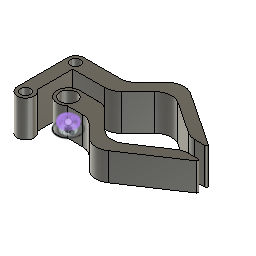
claw (Autodesk Fusion 360 design; units mm, degrees)
Autodesk Fusion 360 part; units mm, degrees
sketch "Sketch1" plane through (0, 0, 0) normal (0, 0, 1) x (1, 0, 0)
  circle A0 centre (0, 0) radius 1.75
  circle A1 centre (1.6986, -0.4211) radius 0.275
  circle A2 centre (0, 0) radius 4
  circle A3 centre (1.723, 0.3062) radius 0.275
  circle A4 centre (1.4495, 0.9805) radius 0.275
  circle A5 centre (0.9254, 1.4853) radius 0.275
  circle A6 centre (0.2412, 1.7333) radius 0.275
  circle A7 centre (-0.4846, 1.6816) radius 0.275
  circle A8 centre (-1.1267, 1.3391) radius 0.275
  circle A9 centre (-1.5739, 0.765) radius 0.275
  circle A10 centre (-1.749, 0.0587) radius 0.275
  circle A11 centre (-1.6217, -0.6577) radius 0.275
  circle A12 centre (-1.214, -1.2605) radius 0.275
  circle A13 centre (-0.5963, -1.6453) radius 0.275
  circle A14 centre (0.1244, -1.7456) radius 0.275
  circle A15 centre (0.8237, -1.5441) radius 0.275
  circle A16 centre (1.3805, -1.0756) radius 0.275
  dimension "d1" = 3.5
  dimension "d2" = 0.55
  dimension "d3" = 8
  dimension "d5" = 360
  constraint coincident A0.centre A2.centre
  constraint coincident A0 A1.centre
  measures "d1" diameter of A0
  measures "d2" diameter of A1
  measures "d3" diameter of A2
extrude "Extrude1" add sketch "Sketch1" along normal blind 2.25 makes body 1
sketch "Sketch2" plane through (0, 0, 2.25) normal (0, 0, 1) x (-1, 0, 0)
  arc A0 (-1.5319, 0.846) -> (-1.6116, 0.682) centre (0, 0) ccw
  arc A1 (-1.1949, 1.2785) -> (-1.5319, 0.846) centre (-1.3805, 1.0756) ccw
  arc A2 (-1.0554, 1.396) -> (-1.1949, 1.2785) centre (0, 0) ccw
  arc A3 (-0.5716, 1.654) -> (-1.0554, 1.396) centre (-0.8237, 1.5441) ccw
  arc A4 (-0.3963, 1.7045) -> (-0.5716, 1.654) centre (0, 0) ccw
  arc A5 (0.1506, 1.7435) -> (-0.3963, 1.7045) centre (-0.1244, 1.7456) ccw
  arc A6 (0.3312, 1.7184) -> (0.1506, 1.7435) centre (0, 0) ccw
  arc A7 (0.8467, 1.5315) -> (0.3312, 1.7184) centre (0.5963, 1.6453) ccw
  arc A8 (1.0015, 1.4351) -> (0.8467, 1.5315) centre (0, 0) ccw
  arc A9 (1.3964, 1.0547) -> (1.0015, 1.4351) centre (1.214, 1.2605) ccw
  arc A10 (1.4986, 0.9037) -> (1.3964, 1.0547) centre (0, 0) ccw
  arc A11 (1.7047, 0.3956) -> (1.4986, 0.9037) centre (1.6217, 0.6577) ccw
  arc A12 (1.7366, 0.216) -> (1.7047, 0.3956) centre (0, 0) ccw
  arc A13 (1.7182, -0.332) -> (1.7366, 0.216) centre (1.749, -0.0587) ccw
  arc A14 (1.6743, -0.509) -> (1.7182, -0.332) centre (0, 0) ccw
  arc A15 (1.4346, -1.0022) -> (1.6743, -0.509) centre (1.5739, -0.765) ccw
  arc A16 (1.3225, -1.146) -> (1.4346, -1.0022) centre (0, 0) ccw
  arc A17 (0.903, -1.499) -> (1.3225, -1.146) centre (1.1267, -1.3391) ccw
  arc A18 (0.7421, -1.5849) -> (0.903, -1.499) centre (0, 0) ccw
  arc A19 (0.2152, -1.7367) -> (0.7421, -1.5849) centre (0.4846, -1.6816) ccw
  arc A20 (0.0333, -1.7497) -> (0.2152, -1.7367) centre (0, 0) ccw
  arc A21 (-0.5098, -1.6741) -> (0.0333, -1.7497) centre (-0.2412, -1.7333) ccw
  arc A22 (-0.6812, -1.612) -> (-0.5098, -1.6741) centre (0, 0) ccw
  arc A23 (-1.1466, -1.322) -> (-0.6812, -1.612) centre (-0.9254, -1.4853) ccw
  arc A24 (-1.278, -1.1955) -> (-1.1466, -1.322) centre (0, 0) ccw
  arc A25 (-1.5852, -0.7414) -> (-1.278, -1.1955) centre (-1.4495, -0.9805) ccw
  arc A26 (-1.6538, -0.5723) -> (-1.5852, -0.7414) centre (0, 0) ccw
  arc A27 (-1.7497, -0.0325) -> (-1.6538, -0.5723) centre (-1.723, -0.3062) ccw
  arc A28 (-1.7436, 0.1498) -> (-1.7497, -0.0325) centre (0, 0) ccw
  arc A29 (-1.6116, 0.682) -> (-1.7436, 0.1498) centre (-1.6986, 0.4211) ccw
  circle A30 centre (0, 0) radius 4
  circle A31 centre (0, 0) radius 1
  dimension "d8" = 2
  measures "d8" diameter of A31
extrude "Extrude2" add sketch "Sketch2" along normal blind 1 contours A0 A1 A2 A3 A4 A5 A6 A7 A8 A9 A10 A11 A12 A13 A14 A15 A16 A17 A18 A19 A20 A21 A22 A23 A24 A25 A26 A27 A28 A29 | A30 bodies 1
sketch "Sketch3" plane through (0, 0, 3.25) normal (0, 0, 1) x (-1, 0, 0)
  circle A0 centre (0, 0) radius 1
  circle A1 centre (0, 0) radius 4
  circle A2 centre (0, 0) radius 3
  line L0 (0, 0) -> (-4, 0) construction
  line L1 (-4, 0) -> (-4, -4) construction
  line L2 (-4, -4) -> (0, -4) construction
  line L3 (0, -4) -> (0, 0) construction
  circle A3 centre (-11.5, -7) radius 7.5
  line L4 (-4, -4) -> (-11.5, -4) construction
  line L5 (-11.5, -4) -> (-11.5, -7) construction
  line L6 (-11.5, -7) -> (-4, -7) construction
  line L7 (-4, -7) -> (-4, -4) construction
  circle A4 centre (-11.5, -7) radius 11
  line L8 (0, -4) -> (-4.6261, -4)
  line L9 (-4.6261, -4) -> (-22.083, -4)
  dimension "d11" = 6
  dimension "d12" = 4
  dimension "d13" = 4
  dimension "d14" = 15
  dimension "d15" = 3
  dimension "d16" = 22
  constraint concentric A0 A2
  constraint horizontal L0
  constraint vertical L1
  constraint horizontal L2
  constraint vertical L3
  constraint coincident A0.centre A1.centre
  constraint horizontal L4
  constraint vertical L5
  constraint horizontal L6
  constraint vertical L7
  constraint coincident A3.centre L5.end
  constraint tangent A3 L7
  constraint concentric A3 A4
  constraint coincident A3 L8.end
  constraint coincident L4 L8.end
  constraint coincident A4 L9.end
  constraint parallel L4 L9
  measures "d11" diameter of A2
  measures "d12" distance of A0.centre L0.end
  measures "d13" distance of A0.centre L2.end
  measures "d14" diameter of A3
  measures "d15" distance of L4.end A3.centre
  measures "d16" diameter of A4
extrude "Extrude3" add sketch "Sketch3" against normal blind 3.25 contours A1 A4 L8 | A1 A3 A4 L8 L9 bodies 1
extrude "Extrude4" add sketch "Sketch3" along normal blind 4.75 contours A1 A2 A4 | A1 A4 L8 | A1 A3 A4 L8 L9 | A1 A2 A4 bodies 1
sketch "Sketch4" plane through (0, 0, 0) normal (0, 0, 1) x (1, 0, 0)
  line L0 (0, 0) -> (-6.35, 0) construction
  line L1 (-6.35, 9) -> (-6.35, -9) construction
  circle A0 centre (-6.35, 9) radius 1.8
  circle A1 centre (-6.35, -9) radius 1.8
  circle A2 centre (-6.35, 9) radius 3
  circle A3 centre (-6.35, -9) radius 3
  line L2 (-4.85, -6.4019) -> (-4.85, 6.4019)
  line L3 (-9.35, -9) -> (-9.35, 9)
  line L4 (11.5, 7) -> (11.5, 5) construction
  circle A4 centre (11.5, 5) radius 7.5
  circle A5 centre (11.5, 5) radius 11
  line L5 (-4.85, 6.4019) -> (22.4103, 6.4019)
  line L6 (-6.35, 12) -> (19.9853, 12)
  point P0 (11.5, 7)
  dimension "d21" = 6.35
  dimension "d22" = 18
  dimension "d23" = 3.6
  dimension "d24" = 3.6
  dimension "d25" = 6
  dimension "d26" = 6
  dimension "d27" = 1.5
  dimension "d28" = 2
  dimension "d29" = 15
  dimension "d30" = 22
  constraint coincident L0.start origin
  constraint horizontal L0
  constraint vertical L1
  constraint midpoint L0.end L1
  constraint coincident L1.start A0.centre
  constraint coincident L1.end A1.centre
  constraint concentric A0 A2
  constraint coincident A3 L2.start
  constraint coincident A2 L2.end
  constraint parallel L1 L2
  constraint vertical L3
  constraint tangent A2 L3
  constraint coincident A3 L3.start
  constraint coincident A2 L3.end
  constraint coincident P0 L4.start
  constraint vertical L4
  constraint coincident L4.end A4.centre
  constraint concentric A4 A5
  constraint coincident A5 L5.end
  constraint perpendicular L2 L5
  constraint horizontal L6
  constraint tangent A2 L6
  constraint coincident A2 L6.start
  constraint coincident A5 L6.end
  measures "d21" distance of L0.start L0.end
  measures "d22" distance of L1.start L1.end
  measures "d23" diameter of A0
  measures "d24" diameter of A1
  measures "d25" diameter of A2
  measures "d26" diameter of A3
  measures "d27" distance of L1 L2
  measures "d28" distance of P0 L4.end
  measures "d29" diameter of A4
  measures "d30" diameter of A5
extrude "Extrude5" add sketch "Sketch4" along normal blind 8 separate body contours A2 | A2 A5 L5 L6 | A2 A3 L2 L3 | A4 A5 L5 L6 | A4 A5 L6 | A3 | A4 A5 L5 L6 makes body 2
extrude "Extrude6" add sketch "Sketch3" along normal blind 0.5 contours A2 A4 picked at (-1.2016, -1.7718) bodies 1
extrude "Extrude7" add 1 faces at (2.2636, 1.3779, 3.25) along direction (0, 0, 1) blind 0.5 on bodies 1 bodies 1
sketch "Sketch5" plane through (0, 0, 8) normal (0, 0, 1) x (-1, 0, 0)
  circle A0 centre (6.35, 9) radius 1.8
  circle A1 centre (6.35, -9) radius 1.8
  arc A2 (9.35, 9) -> (4.85, 6.4019) centre (6.35, 9) ccw
  line L0 (4.85, 6.4019) -> (4.85, -6.4019)
  line L1 (4.85, -6.4019) -> (-4.1322, -6.4019)
  arc A3 (-18.8678, -6.4019) -> (-4.1322, -6.4019) centre (-11.5, -5) ccw
  line L2 (-18.8678, -6.4019) -> (-22.4103, -6.4019)
  arc A4 (-22.4103, -6.4019) -> (-3.0147, -12) centre (-11.5, -5) ccw
  line L3 (-3.0147, -12) -> (6.35, -12)
  arc A5 (6.35, -12) -> (9.35, -9) centre (6.35, -9) ccw
  line L4 (9.35, -9) -> (9.35, 9)
  line L5 (-4.1322, -6.4019) -> (-9.1322, -6.4019)
  line L6 (-9.1322, -6.4019) -> (-20.3752, -17.6449)
  line L7 (-3.4753, -6.4019) -> (-20.3752, -23.3018)
  line L8 (-3.0147, -12) -> (-33.8385, -12) construction
  line L9 (-20.3752, -17.6449) -> (-37.275, -6.4019)
  line L10 (-3.4753, -6.4019) -> (-56.0388, -6.4019) construction
  line L11 (-23.2036, -20.4733) -> (-44.355, -6.4019)
  line L12 (-20.3752, -17.6449) -> (-23.2036, -20.4733)
  line L13 (-37.275, -6.4019) -> (-44.355, -6.4019)
  line L14 (-23.2036, -20.4733) -> (-16.745, -24.7701)
  line L15 (-3.0147, -12) -> (-9.0734, -12)
  line L16 (-9.1322, -6.4019) -> (-24.5268, -6.4019) construction
  line L17 (-24.5268, -6.4019) -> (-24.5268, -5.2009) construction
  line L18 (-24.5268, -5.2009) -> (-9.1322, -5.2009) construction
  line L19 (-9.1322, -5.2009) -> (-9.1322, -6.4019) construction
  line L20 (-9.1322, -3.9999) -> (-20.3752, 7.2431)
  line L21 (-20.3752, 7.2431) -> (-23.2036, 10.0715)
  line L22 (-23.2036, 10.0715) -> (-44.355, -3.9999)
  line L23 (-3.4753, -3.9999) -> (-20.3752, 12.8999)
  line L24 (-23.2036, 10.0715) -> (-16.745, 14.3682)
  line L25 (-20.3752, 7.2431) -> (-37.275, -3.9999)
  line L26 (-37.275, -3.9999) -> (-44.355, -3.9999)
  line L27 (-4.1322, -3.9999) -> (-9.1322, -3.9999)
  line L28 (-4.1322, -3.9999) -> (-3.4753, -3.9999)
  dimension "d37" = 5
  dimension "d38" = 15.9
  dimension "d40" = 135
  dimension "d44" = 1.201
  constraint coincident L1.end A3.end
  constraint parallel L1 L5
  constraint coincident A4.end L3.start
  constraint horizontal L8
  constraint horizontal L10
  constraint coincident L10 L11.end
  constraint parallel L9 L11
  constraint coincident L11 L12.end
  constraint parallel L11 L14
  constraint coincident L7 L15.end
  constraint coincident L8 L15.end
  constraint parallel L6 L7
  constraint horizontal L16
  constraint vertical L17
  constraint horizontal L18
  constraint vertical L19
  constraint symmetric L1.end L18 L27.start
  constraint symmetric L5.end L18 L20.start
  constraint symmetric L6.end L18 L20.end
  constraint symmetric L7.start L18 L23.start
  constraint symmetric L7.end L18 L23.end
  constraint symmetric L9.end L18 L25.end
  constraint symmetric L11.start L18 L21.end
  constraint symmetric L11.end L18 L22.end
  constraint symmetric L14.end L18 L24.end
  constraint parallel L27 L28
  measures "d37" distance of L1.end L5.end
  measures "d38" distance of L5.end L6.end
  measures "d40" angle of L5 L6
  measures "d44" distance of L5.end L18.end
extrude "Extrude8" cut sketch "Sketch5" against normal blind 8 contours A3 A4 L7 L15 | A3 A4 L6 L7 | A3 L2 A4 L6 bodies 2
sketch "Sketch6" plane through (0, 0, 8) normal (0, 0, 1) x (-1, 0, 0)
  circle A0 centre (0, 0) radius 3
  arc A1 (0, -4) -> (-3.8878, 0.9407) centre (0, 0) ccw
  arc A2 (-3.8878, 0.9407) -> (-22.083, -4) centre (-11.5, -7) ccw
  line L0 (-22.083, -4) -> (-18.3739, -4)
  arc A3 (-4.6261, -4) -> (-18.3739, -4) centre (-11.5, -7) ccw
  line L1 (-4.6261, -4) -> (0, -4)
  line L2 (-3.4753, -3.9999) -> (-20.3752, 12.8999)
  line L3 (0, 3) -> (-10.4753, 3)
  line L4 (-13.3901, 0.2579) -> (-16.1165, 2.9844)
  constraint coincident A0 L3.start
  constraint coincident L2 L3.end
  constraint tangent A0 L3
  constraint horizontal L3
  constraint coincident A3 L4.start
  constraint coincident A2 L4.end
extrude "Extrude9" cut sketch "Sketch6" against normal blind 8 contours A2 L0 A3 L4 bodies 1
extrude "Extrude10" add sketch "Sketch5" sketch "Sketch6" against normal blind 8 contours L20 L21 L23 L24 L27 L28 of sketch 2 contours A1 A2 L3 bodies 1
extrude "Extrude11" cut sketch "Sketch6" against normal blind 8 contours A2 L2 L3 bodies 1
extrude "Extrude12" add sketch "Sketch5" against normal blind 8 contours L21 L22 L25 L26 bodies 1
extrude "Extrude13" add sketch "Sketch5" against normal blind 8 contours A3 L5 L6 L7 | A3 L7 L15 | A4 L6 L7 L12 L14 | A3 A4 L6 L7 | L9 L11 L12 L13 picked at (-6.0677, -9.2001) bodies 2
fillet "Fillet1" radius 6 10 edges at (19.8067, -12.3314, 4) (10.4753, -3, 4) (20.3752, -7.2431, 4) (9.1322, 3.9999, 4) (37.275, 3.9999, 4) (37.275, 6.4019, 4) (20.3752, 17.6449, 4) (9.1322, 6.4019, 4) (19.8067, 22.7332, 4) (9.0734, 12, 4) on bodies 1 2
fillet "Fillet2" radius 0.5 2 edges at (44.355, 3.9999, 4) (44.355, 6.4019, 4) on bodies 1 2
extrude "Extrude14" add 2 faces at (2.895, 9.134, 8) (34.2136, -1.1768, 8) along direction (0, 0, 1) blind 2 on bodies 1 2 bodies 2 1
extrude "Extrude15" add 1 faces at (2.895, 9.134, 10) along direction (0, 0, 1) blind 3 on bodies 2 bodies 2
